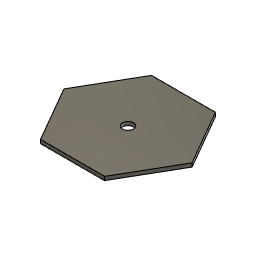
BottomTest v4 (Autodesk Fusion 360 design; units mm, degrees)
Autodesk Fusion 360 part; units mm, degrees
sketch "草图1" plane through (0, 0, 0) normal (0, 1, 0) x (1, 0, 0)
  line L0 (70, 0) -> (35, 60.6218)
  line L1 (35, 60.6218) -> (-35, 60.6218)
  line L2 (-35, 60.6218) -> (-70, 0)
  line L3 (-70, 0) -> (-35, -60.6218)
  line L4 (-35, -60.6218) -> (35, -60.6218)
  line L5 (35, -60.6218) -> (70, 0)
  dimension "d1" = 70
  measures "d1" distance of origin L0.start
extrude "拉伸1" add sketch "草图1" along normal blind 4
hole "孔1" at (0, 4, 0) direction (0, -1, 0) diameter 12 depth 30 tip angle 180
